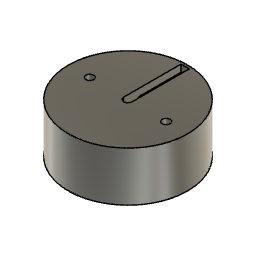
RETHI Hex Screwdriver Mount Cap (Autodesk Fusion 360 design; units mm, degrees)
Autodesk Fusion 360 part; units mm, degrees
sketch "Sketch2" plane through (0, 0, 0) normal (0, 0, 1) x (1, 0, 0)
  circle A0 centre (0, 0) radius 26.5
  dimension "diam" = 53
  constraint coincident A0.centre origin
  measures "diam" diameter of A0
extrude "Extrude1" add sketch "Sketch2" along normal blind 22 makes body 1
ref_plane "WorkPlane1" through (-26.5, 0, 42.6906) normal (-1, 0, 0) x (0, 1, 0)
ref_plane "WorkPlane2" through (0, 0, 42.6906) normal (-1, 0, 0) x (0, 1, 0)
sketch "Sketch3" plane through (0, 0, 102.2963) normal (-1, 0, 0) x (0, 1, 0)
  line L0 (0, 80.2963) -> (0, 181.8963)
  line L1 (0, 80.2963) -> (25.4, 80.2963)
  line L2 (-26.5, 80.2963) -> (26.5, 80.2963)
  line L3 (-26.5, 80.2963) -> (26.5, 80.2963)
  point P0 (0, 80.2963)
  dimension "armLength" = 101.6
  dimension "armWidth" = 25.4
  constraint vertical L0
  constraint perpendicular L0 L1
  constraint coincident P0 L0
  constraint coincident P0 L1
  constraint coincident P0 L2
  constraint midpoint P0 L3
  constraint coincident P0 L0.start
  measures "armLength" distance of P0 L0.end
  measures "armWidth" distance of P0 L1.end
ref_plane "WorkPlane6" through (0, 26.5, 5.9315) normal (0, 1, 0) x (1, 0, 0)
ref_plane "WorkPlane7" through (0, 25.4, 5.9315) normal (0, 1, 0) x (1, 0, 0)
sketch "Sketch6" plane through (0, 25.4, 14.2132) normal (0, 1, 0) x (1, 0, 0)
  line L0 (1.8331, -4.6118) -> (1.8331, -7.7868)
  line L1 (-1.8331, -7.7868) -> (-1.8331, -4.6118)
  line L2 (1.8331, -7.7868) -> (-1.8331, -7.7868)
  line L3 (-1.8331, -4.6118) -> (1.8331, -4.6118)
  point P0 (0, -7.7868)
  dimension "d187" = 3.175
  constraint vertical L0
  constraint perpendicular L1 L2
  constraint perpendicular L0 L3
  measures "d187" distance of L1.start L1.end
sketch "Sketch1" plane through (0, 0, 0) normal (0, 0, 1) x (1, 0, 0) in component "Cap"
  circle A0 centre (127, 0.0001) radius 26.5
  circle A1 centre (127, -16.9749) radius 5.125
  circle A2 centre (127, 16.9751) radius 5.125
  circle A3 centre (127, 16.9751) radius 1.7272
  circle A4 centre (127, -16.9749) radius 1.7272
  line L0 (127, -16.9749) -> (127, 16.9751)
  dimension "d69" = 53
  dimension "d81" = 10.25
  dimension "d82" = 10.25
  dimension "d85" = 33.95
  dimension "d143" = 3.4544
  dimension "d144" = 3.4544
  constraint concentric A2 A3
  constraint concentric A1 A4
  constraint coincident A1.centre A4.centre
  constraint coincident A2.centre A3.centre
  constraint vertical L0
  constraint midpoint A0.centre L0
  measures "d69" diameter of A0
  measures "d81" diameter of A1
  measures "d82" diameter of A2
  measures "d85" distance of A1.centre A2.centre
  measures "d143" diameter of A3
  measures "d144" diameter of A4
extrude "Extrude1'" add sketch "Sketch1" along normal blind 5.02 separate body contours A0 | A1 | A2 makes body 2 in component "Cap"
ref_plane "WorkPlane1" through (153.5, 0.0001, 15.298) normal (1, 0, 0) x (0, -1, 0) in component "Cap"
ref_plane "WorkPlane4" through (152.4, 0.0001, 15.298) normal (1, 0, 0) x (0, -1, 0) in component "Cap"
sketch "Sketch4" plane through (152.4, 0, 21.9945) normal (1, 0, 0) x (0, 1, 0) in component "Cap"
  line L0 (26.5001, -16.9745) -> (-26.4999, -16.9745)
  line L1 (0.0001, -16.9745) -> (0.0001, -18.562)
  line L2 (-1.833, -16.9745) -> (1.8331, -16.9745)
  line L3 (-0.9165, -18.562) -> (0.9166, -18.562)
  line L4 (0.9166, -18.562) -> (1.8331, -16.9745)
  line L5 (-1.833, -16.9745) -> (-0.9165, -18.562)
  line L6 (-1.833, -16.9745) -> (1.8331, -16.9745)
  line L7 (-18.7021, -16.9745) -> (-15.2477, -16.9745)
  line L8 (15.2479, -16.9745) -> (18.7023, -16.9745)
  dimension "d76" = 1.5875
  dimension "d77" = 120
  dimension "d78" = 120
  constraint midpoint L0 L1.start
  constraint perpendicular L0 L1
  constraint coincident L0 L2.start
  constraint coincident L0 L2.end
  constraint horizontal L3
  constraint equal L3 L5
  constraint midpoint L1.end L3
  measures "d76" distance of L1.start L1.end
  measures "d77" angle of L3 L5
  measures "d78" angle of L3 L4
sketch "Sketch7" plane through (0, 0, 22) normal (0, 0, 1) x (-1, 0, 0)
  circle A0 centre (0, 0) radius 26.5
  circle A1 centre (-16.9749, 0) radius 1.7272
  line L0 (16.9749, 0) -> (-16.9749, 0)
  circle A2 centre (16.9751, 0) radius 1.7272
  circle A3 centre (-16.9749, 0) radius 3.585
  circle A4 centre (16.9749, 0) radius 3.585
  dimension "d152" = 33.95
  dimension "d153" = 3.4544
  dimension "d154" = 3.4544
  dimension "d156" = 7.17
  dimension "d157" = 7.17
  constraint coincident A1.centre L0.end
  constraint midpoint A0.centre L0
  constraint coincident L0.start A4.centre
  measures "d152" distance of A1.centre A2.centre
  measures "d153" diameter of A1
  measures "d154" diameter of A2
  measures "d156" diameter of A3
  measures "d157" diameter of A4
extrude "Extrude3" cut sketch "Sketch7" against normal blind 8 contours A1 | A2 bodies 1
sketch "Sketch6 (2)" plane through (0, 0, 0) normal (0, 0, -1) x (1, 0, 0) in component "Cap"
  circle A0 centre (127, -0.0001) radius 26.5
  circle A1 centre (127, -0.0001) radius 8.8333
  circle A2 centre (127, 16.9749) radius 1.7272
  circle A3 centre (127, -16.9751) radius 1.7272
  circle A4 centre (127, -0.0001) radius 3
  dimension "d105" = 17.6667
  dimension "d190" = 6
  constraint concentric A0 A1
  constraint concentric A1 A4
  measures "d105" diameter of A1
  measures "d190" diameter of A4
extrude "Extrude4" add sketch "Sketch6 (2)" along normal blind 19.1861 contours A1 | A4 bodies 2 in component "Cap"
sketch "Sketch10" plane through (0, 0, 0) normal (0, 0, -1) x (1, 0, 0)
  circle A0 centre (0, 0) radius 26.5
  circle A1 centre (0, 0) radius 18.5
  dimension "bearingDiam" = 37
  constraint coincident A0.centre A1.centre
  measures "bearingDiam" diameter of A1
extrude "Extrude4'" cut sketch "Sketch10" against normal blind 12.0396 contours A1 bodies 1
extrude "Extrude9" cut sketch "Sketch6 (2)" along normal up to surface (19.1861 mm away) and the other way blind 0 contours A4 bodies 2 in component "Cap"
sketch "Sketch12" plane through (0, 0, 22) normal (0, 0, 1) x (-1, 0, 0)
  circle A0 centre (0, 0) radius 26.5
  circle A1 centre (0, 0) radius 1.8331
  circle A2 centre (-16.9749, 0) radius 1.7272
  circle A3 centre (16.9751, 0) radius 1.7272
  constraint concentric A0 A1
extrude "Extrude6" cut sketch "Sketch12" against normal up to surface (9.9604 mm away) contours A1 bodies 1
extrude "Extrude7" cut sketch "Sketch6" along normal blind 0 and the other way blind 25.5 bodies 1
move_body "Move1" bodies 2 to x (1, 0, 0) y (0, -1, 0) z (0, 0, -1) at (0, -27.5999, 38.1) in component "Cap"
move_body "Move2" bodies 2 to x (0, 1, 0) y (-1, 0, 0) z (0, 0, 1) at (-56.5474, -223.8853, -59.5692) in component "Cap"
fillet "Fillet2" radius 5 1 edges at (-32.1417, -105.1209, -21.4692) on bodies 2 in component "Cap"
ref_plane "WorkPlane6" through (-37.7808, -96.8853, 9.4824) normal (-1, 0, 0) x (0, 1, 0) in component "Cap"
sketch "Sketch12 (2)" plane through (-37.7808, -96.8853, 9.4824) normal (-1, 0, 0) x (0, 1, 0) in component "Cap"
  circle A0 centre (0, 15.3735) radius 1.25
  line L0 (0, 15.3735) -> (0, 22.2315)
  circle A1 centre (0, 22.2315) radius 1.25
  circle A2 centre (0, 22.2315) radius 3.25
  circle A3 centre (0, 15.3735) radius 3.25
  line L1 (-8.8333, 11.7655) -> (8.8333, 11.7655)
  line L2 (0, 23.4815) -> (-1.524, 23.4815)
  dimension "d196" = 2.5
  dimension "d198" = 2.5
  dimension "d207" = 6.5
  dimension "d208" = 6.5
  dimension "d218" = 13.716
  dimension "d219" = 6.858
  constraint coincident A0.centre L0.start
  constraint vertical L0
  constraint coincident L0.end A1.centre
  constraint concentric A1 A2
  constraint coincident A1 L2.start
  constraint tangent A1 L2
  constraint horizontal L2
  measures "d196" diameter of A0
  measures "d198" diameter of A1
  measures "d207" diameter of A2
  measures "d208" diameter of A3
  measures "d219" distance of A0.centre L0.end
sketch "Sketch9" plane through (0, 0, -21.4692) normal (0, 0, 1) x (-1, 0, 0) in component "Cap"
  circle A0 centre (11.9724, 96.8853) radius 1.7272
  circle A1 centre (28.9474, 96.8853) radius 26.5
  circle A2 centre (45.9224, 96.8853) radius 1.7272
  circle A3 centre (45.9224, 96.8853) radius 5.15
  circle A4 centre (11.9724, 96.8853) radius 5.15
  line L0 (45.9224, 96.8853) -> (11.9725, 96.8853)
  circle A5 centre (28.9474, 96.8853) radius 13.8333
  dimension "d145" = 10.3
  dimension "d146" = 10.3
  dimension "d147" = 33.95
  constraint coincident A2.centre A3.centre
  constraint concentric A2 A3
  measures "d145" diameter of A3
  measures "d146" diameter of A4
  measures "d147" distance of A0.centre A2.centre
extrude "Extrude10" cut sketch "Sketch12 (2)" along normal up to surface contours A0 | A1 end surface at (-31.8353, -96.0728, -8.6785) on bodies 2 bodies 2 in component "Cap"
extrude "Extrude5" [suppressed]
fillet "Fillet4" [suppressed]
extrude "Extrude11" cut sketch "Sketch12 (2)" against normal blind 1.7 draft -45 contours A0 | A1 | A2 | A3 bodies 2 in component "Cap"
sketch "Sketch13" plane through (0, 0, 18.825) normal (0, 0, 1) x (-1, 0, 0)
  line L0 (-1.8331, 0) -> (-1.8331, -25.4)
  line L1 (1.8331, -25.4) -> (1.8331, 0)
  line L2 (-1.8331, -6) -> (1.8331, -6)
  line L3 (1.8331, -6) -> (1.8331, 0)
  line L4 (1.8331, 0) -> (-1.8331, 0)
  line L5 (-1.8331, 0) -> (-1.8331, -6)
  arc A0 (-1.8331, 0) -> (1.8331, 0) centre (0, 0) ccw
  line L6 (-1.8331, -25.4) -> (1.8331, -25.4)
  dimension "d211" = 6
  constraint horizontal L2
  constraint vertical L3
  constraint horizontal L4
  constraint vertical L5
  constraint coincident L1.end L3.end
  constraint coincident L0 L2.start
  measures "d211" distance of L2.end L1.end
extrude "Extrude8" cut sketch "Sketch13" against normal blind 4 contours L0 L1 L2 L3 L5 A0 bodies 1
fillet "Fillet5" radius 1 2 edges at (0, 6, 18.825) (0, 1.8331, 14.825) on bodies 1
component "Cap" placed x (1, 0, 0) y (0, 1, 0) z (0, 0, 1) at (28.9474, 96.8853, 48.4892)
equation "d5 = ( -diam / 2 )"
equation "d12 = -( ( diam / 2 ) - 1 in )"
equation "hexDiam = 0.125 in"
equation "d69 = diam"
equation "d70 = 0.25 in - 1.33 mm"
equation "d75 = -( ( diam / 2 ) - 1 in )"
equation "d76 = hexDiam / 2"
equation "d85 = diam - 0.75 in"
equation "motorShaftDiam = 0.125 in"
equation "motorShaftLength = 0.953 in - 0.19764 in"
equation "d105 = diam / 3"
equation "d108 = motorShaftLength"
equation "chamberTrack = 0.474 in"
equation "d147 = diam - 0.75 in"
equation "d152 = diam - 0.75 in"
equation "d187 = 1.5875 * 2 mm"
